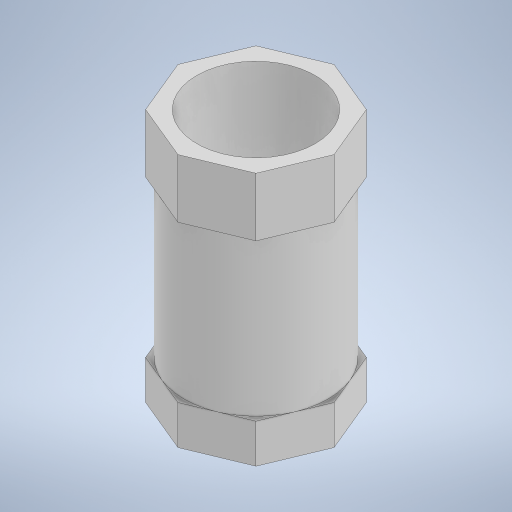
# Autodesk Inventor part: TUBO_METALICO_B
Saved by Autodesk Inventor 2024 (Build 280153000, 153)
## iProperties
Created: 2022-10-31
Part Number: TUBO_METALICO_B
Material: Genérico
Document SubType Name: Modeling
Designer: Usuario
Density: 1 g/cm^3
Appearance: Valor por defecto
Author: Usuario
Autodesk Inventor part; units mm, degrees
ref_plane "YZ Plane" through (0, 0, 0) normal (1, 0, 0) x (0, 1, 0)
ref_plane "XZ Plane" through (0, 0, 0) normal (0, 1, 0) x (-1, 0, 0)
ref_plane "XY Plane" through (0, 0, 0) normal (0, 0, 1) x (1, 0, 0)
sketch "Boceto1" plane through (0, 0, 0) normal (0, 1, 0) x (-1, 0, 0)
  circle A0 centre (0, 0) radius 10
  line L0 (7.0711, -7.0711) -> (0, -10)
  line L1 (10, 0) -> (7.0711, -7.0711)
  line L2 (0, -10) -> (-7.0711, -7.0711)
  line L3 (-10, 0) -> (-7.0711, -7.0711)
  line L4 (0, 10) -> (7.0711, 7.0711)
  line L5 (7.0711, 7.0711) -> (10, 0)
  line L6 (0, 0) -> (0, 10)
  line L7 (0, 10) -> (-7.0711, 7.0711)
  line L8 (-7.0711, 7.0711) -> (-10, 0)
  circle A1 centre (0, 0) radius 10
  line L9 (7.0711, -7.0711) -> (0, -10)
  line L10 (10, 0) -> (7.0711, -7.0711)
  line L11 (0, -10) -> (-7.0711, -7.0711)
  line L12 (-10, 0) -> (-7.0711, -7.0711)
  line L13 (0, 10) -> (7.0711, 7.0711)
  line L14 (7.0711, 7.0711) -> (10, 0)
  line L15 (0, 0) -> (0, 10)
  line L16 (-7.0711, 7.0711) -> (-10, 0)
  line L17 (0, 10) -> (-7.0711, 7.0711)
  dimension "d0" = 20
  dimension "d5" = 20
  constraints: 36 end point, 4 symmetric about line, 2 coincident, 2 parallel, 2 vertical, 22 other
extrude "Extrusión1" add sketch "Boceto1" along normal blind 5 contours L1 L0 L2 L3 L8 L7 L4 L5
sketch "Boceto2" plane through (0, 5, 0) normal (0, 1, 0) x (1, 0, 0)
  circle A0 centre (0, 0) radius 9.2388
  line L0 (0, 10) -> (-7.0711, 7.0711) projected
  constraints: 1 centre point, 1 coincident, 1 tangent
extrude "Extrusión2" add sketch "Boceto2" along normal blind 20
sketch "Boceto3" plane through (0, 25, 0) normal (0, 1, 0) x (1, 0, 0)
  line L0 (7.0711, -7.0711) -> (8.5355, -3.5355) projected
  line L1 (8.5355, -3.5355) -> (10, 0) projected
  line L2 (10, 0) -> (8.5355, 3.5355) projected
  line L3 (8.5355, 3.5355) -> (7.0711, 7.0711) projected
  line L4 (7.0711, 7.0711) -> (3.5355, 8.5355) projected
  line L5 (3.5355, 8.5355) -> (0, 10) projected
  line L6 (0, -10) -> (3.5355, -8.5355) projected
  line L7 (3.5355, -8.5355) -> (7.0711, -7.0711) projected
  line L8 (0, -10) -> (7.0711, -7.0711)
  line L9 (7.0711, -7.0711) -> (10, 0) projected
  line L10 (10, 0) -> (7.0711, 7.0711) projected
  line L11 (10, 0) -> (7.0711, 7.0711)
  line L12 (7.0711, 7.0711) -> (0, 10)
  line L13 (0, 0) -> (0, 10)
  line L14 (-7.0711, -7.0711) -> (-8.5355, -3.5355)
  line L15 (-8.5355, -3.5355) -> (-10, 0)
  line L16 (-10, 0) -> (-8.5355, 3.5355)
  line L17 (-8.5355, 3.5355) -> (-7.0711, 7.0711)
  line L18 (-7.0711, 7.0711) -> (-3.5355, 8.5355)
  line L19 (-3.5355, 8.5355) -> (0, 10)
  line L20 (0, -10) -> (-3.5355, -8.5355)
  line L21 (-3.5355, -8.5355) -> (-7.0711, -7.0711)
  line L22 (0, -10) -> (-7.0711, -7.0711)
  line L23 (-7.0711, -7.0711) -> (-10, 0)
  line L24 (-10, 0) -> (-7.0711, 7.0711)
  line L25 (-10, 0) -> (-7.0711, 7.0711)
  line L26 (-7.0711, 7.0711) -> (0, 10)
  constraints: 34 end point, 7 symmetric about line, 2 collinear, 1 vertical
extrude "Extrusión3" add sketch "Boceto3" along normal blind 7.5
sketch "Boceto4" plane through (0, 32.5, 0) normal (0, 1, 0) x (1, 0, 0)
  point P0 (0, 0)
  point P1 (0, 0)
  constraints: 1 coincident
hole "Agujero1" at (0, 32.5, 0) direction (0, -1, 0) diameter 15.1638 end through all thread size "11/16-12 UN" class "2B" standard "ANSI Unified Screw Threads"
scale "Escala1" factors (0.2666666, 0.2666666, 0.2666666) then translate (0, 11.9167, 0) bodies 1
